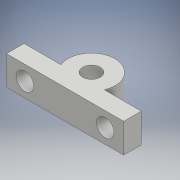
# Autodesk Inventor part: Mount for exis
Saved by Autodesk Inventor 2018 (Build 220112000, 112)
## iProperties
Created: 2019-04-02
Part Number: Mount for exis
Material: Типовые
Document SubType Name: Modeling
Designer: cosko
Density: 1 g/cm^3
Appearance: По умолчанию
Author: cosko
Autodesk Inventor part; units mm, degrees
ref_plane "YZ Plane" through (0, 0, 0) normal (1, 0, 0) x (0, 1, 0)
ref_plane "XZ Plane" through (0, 0, 0) normal (0, 1, 0) x (-1, 0, 0)
ref_plane "XY Plane" through (0, 0, 0) normal (0, 0, 1) x (1, 0, 0)
sketch "Эскиз1" plane through (0, 0, 0) normal (0, 0, 1) x (1, 0, 0)
  line L0 (0, 0) -> (0, 3) construction
  line L1 (0, 3) -> (2.6556, 3) construction
  line L2 (0, 3) -> (0, 6) construction
  circle A0 centre (0, 4.5) radius 1.5
  circle A1 centre (0, 4.5) radius 4
  line L3 (-10, 0) -> (10, 0)
  line L4 (10, 0) -> (10, 3)
  line L5 (10, 3) -> (-10, 3)
  line L6 (-10, 3) -> (-10, 0)
  line L7 (-10, 0) -> (10, 3) construction
  line L8 (10, 0) -> (-10, 3) construction
  point P0 (0, 1.5)
  dimension "d0" = 3
  dimension "d1" = 3
  dimension "d2" = 2.5
  dimension "d3" = 20
  dimension "d4" = 3
  constraints: 18 end point, 4 midpoint, 2 horizontal, 2 parallel, 2 vertical, 1 centre point, 1 perpendicular, 1 vertical alignment, 2 other
  measures "d0" distance of L0.start L0.end
  measures "d1" distance of L0.end L2.end
  measures "d3" distance of L5.end L4.end
  measures "d4" distance of L4.end L3.end
extrude "Выдавливание1" add sketch "Эскиз1" along normal blind 5
sketch "Эскиз4" plane through (3.7081, 3, 0) normal (0, 1, 0) x (1, 0, 0)
  line L0 (0, -5) -> (0, 0) projected
  line L1 (6.2919, -5) -> (0, -5) projected
  line L2 (6.2919, 0) -> (6.2919, -5) projected
  line L3 (6.2919, 0) -> (0, 0) projected
  line L4 (-7.4162, 0) -> (-7.4162, -5) projected
  line L5 (-7.4162, 0) -> (-13.7081, 0) projected
  line L6 (-13.7081, 0) -> (-13.7081, -5) projected
  line L7 (-7.4162, -5) -> (-13.7081, -5) projected
  line L8 (6.2919, -5) -> (0, -5) construction
  line L9 (3.146, -5) -> (3.146, 0) construction
  line L10 (-13.7081, -5) -> (6.2919, -5) construction
  line L11 (-10.5621, -5) -> (-10.5621, 0) construction
  line L12 (-13.7081, 0) -> (6.2919, 0) construction
  circle A0 centre (3.146, -2.5) radius 1.5
  circle A1 centre (-10.5621, -2.5) radius 1.5
  point P0 (-3.7081, 0)
  dimension "d14" = 3
  dimension "d15" = 3
  constraints: 4 end point, 4 midpoint, 2 centre point, 2 point on line, 1 parallel
  measures "d14" diameter of A0
  measures "d15" diameter of A1
extrude "Выдавливание4" cut sketch "Эскиз4" against normal blind 10 contours A0 | A1
